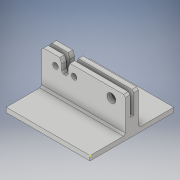
# Autodesk Inventor part: Part3
Saved by Autodesk Inventor 2019 (Build 230136000, 136)
## iProperties
Created: 2018-10-26
Part Number: Part3
Material: Generic
Document SubType Name: Modeling
Designer: Steven
Density: 1 g/cm^3
Appearance: Default
Author: Steven
Autodesk Inventor part; units mm, degrees
ref_plane "YZ Plane" through (0, 0, 0) normal (1, 0, 0) x (0, 1, 0)
ref_plane "XZ Plane" through (0, 0, 0) normal (0, 1, 0) x (-1, 0, 0)
ref_plane "XY Plane" through (0, 0, 0) normal (0, 0, 1) x (1, 0, 0)
sketch "Sketch1" plane through (0, 0, 0) normal (0, 1, 0) x (-1, 0, 0)
  line L0 (0, 0) -> (90, 0)
  line L1 (90, 0) -> (90, -90)
  line L2 (90, -90) -> (0, -90)
  line L3 (0, -90) -> (0, 0)
  dimension "d0" = 90
  dimension "d1" = 90
  constraints: 8 end point, 2 parallel, 1 horizontal, 1 perpendicular
  measures "d0" distance of L1.end L2.end
  measures "d1" distance of L0.end L1.end
extrude "Extrusion1" add sketch "Sketch1" along normal blind 5
sketch "Sketch2" plane through (0, 5, 0) normal (0, 1, 0) x (1, 0, 0)
  line L0 (-90, 90) -> (-90, 0) construction
  line L1 (-90, 45) -> (0, 45) construction
  line L2 (0, 0) -> (0, 90) construction
  line L3 (-90, 43) -> (0, 43)
  line L4 (0, 43) -> (0, 38)
  line L5 (0, 38) -> (-90, 38)
  line L6 (-90, 38) -> (-90, 43)
  line L7 (-90, 47) -> (0, 47)
  line L8 (0, 47) -> (0, 52)
  line L9 (0, 52) -> (-90, 52)
  line L10 (-90, 52) -> (-90, 47)
  dimension "d5" = 5
  dimension "d6" = 5
  dimension "d7" = 2
  dimension "d8" = 2
  constraints: 18 end point, 4 parallel, 4 point on line, 2 horizontal, 2 midpoint, 2 perpendicular
  measures "d5" distance of L3.end L4.end
  measures "d6" distance of L8.end L7.end
  measures "d7" distance between parallel lines of L3 L1
  measures "d8" distance between parallel lines of L7 L1
extrude "Extrusion2" add sketch "Sketch2" along normal blind 37
sketch "Sketch3" plane through (-90, 5, -38) normal (0, 0, 1) x (1, 0, 0)
  circle A0 centre (15, 27) radius 3
  circle A1 centre (35, 27) radius 3
  circle A2 centre (75, 27) radius 4.75
  line L0 (0, 0) -> (0, 37) projected
  line L1 (90, 0) -> (90, 37) projected
  line L2 (0, 37) -> (90, 37) projected
  line L3 (28.5, 25.5503) -> (26.4497, 23.5)
  line L4 (26.4497, 23.5) -> (23.5503, 23.5)
  line L5 (23.5503, 23.5) -> (21.5, 25.5503)
  line L6 (21.5, 25.5503) -> (28.5, 25.5503)
  point P0 (90, -5)
  point P1 (25, 27)
  point P2 (25, 27)
  dimension "d11" = 6
  dimension "d12" = 6
  dimension "d13" = 9.5
  dimension "d14" = 20
  dimension "d15" = 40
  dimension "d16" = 15
  dimension "d17" = 15
  dimension "d18" = 10
  dimension "d20" = 10
  constraints: 8 end point, 3 centre point, 1 coincident, 6 other
  measures "d11" diameter of A0
  measures "d12" diameter of A1
  measures "d13" diameter of A2
  measures "d14" distance of A1.centre A0.centre
  measures "d15" distance of A2.centre A1.centre
  measures "d16" distance from line of L0 A0.centre
  measures "d17" distance from line of L1 A2.centre
  measures "d18" distance from line of A0.centre L2
  measures "d20" distance of point (25, 27) A1.centre
extrude "Extrusion3" cut sketch "Sketch3" against normal blind 14
sketch "Sketch4" plane through (-90, 5, -38) normal (0, 0, 1) x (1, 0, 0)
  line L0 (21.5, 25.5503) -> (28.5, 25.5503) projected
  line L1 (90, 37) -> (0, 37) projected
  line L2 (21.5, 25.5503) -> (28.5, 25.5503)
  line L3 (28.5, 25.5503) -> (28.5, 37)
  line L4 (28.5, 37) -> (21.5, 37)
  line L5 (21.5, 37) -> (21.5, 25.5503)
  point P0 (90, -5)
  dimension "d24" = 7
  constraints: 8 end point, 2 parallel, 1 horizontal, 1 perpendicular, 1 point on line
  measures "d24" distance of L4.end L3.end
extrude "Extrusion4" cut sketch "Sketch4" against normal blind 14
sketch "Sketch5" plane through (0, 5, 0) normal (0, 1, 0) x (1, 0, 0)
  point P0 (0, 0)
sketch "Sketch6" plane through (0, 5, 0) normal (0, 1, 0) x (1, 0, 0)
  line L0 (-90, 47) -> (-90, 43) projected
  line L1 (0, 43) -> (0, 47) projected
  line L2 (-90, 43) -> (0, 43)
  line L3 (0, 43) -> (0, 47)
  line L4 (0, 47) -> (-90, 47)
  line L5 (-90, 47) -> (-90, 43)
  point P0 (0, 0)
  constraints: 8 end point, 2 parallel, 1 horizontal, 1 perpendicular
extrude "Extrusion5" add sketch "Sketch6" along normal blind 14
chamfer "Chamfer1" distance 2 angle 45 6 edges at (-45, 5, -52) (0, 42, -40.5) (0, 42, -49.5) (-90, 42, -49.5) (-90, 42, -40.5) (-45, 5, -38)
chamfer "Chamfer2" distance 2 distance2 5 1 edges at (-68.5, 42, -40.5) measured on face at (-81.5, 42, -41.3333)
chamfer "Chamfer3" distance 2 distance2 5 1 edges at (-68.5, 42, -49.5) measured on face at (-81.5, 42, -50.3333)
chamfer "Chamfer4" distance 2 distance2 5 1 edges at (-61.5, 42, -49.5) measured on face at (-21.8333, 42, -48.6667)
chamfer "Chamfer5" distance 2 distance2 5 1 edges at (-61.5, 42, -40.5) measured on face at (-41.6667, 42, -41.3333)
body "Solid1"
